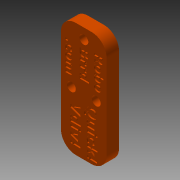
# Autodesk Inventor part: quickvdiv_v1
Saved by Autodesk Inventor 2014 SP1 (Build 180222100, 222)
## iProperties
Created: 2014-02-28
Part Number: quickvdiv_v1
Material: Generic
Document SubType Name: Modeling
Designer: Erin
Density: 1 g/cm^3
Appearance: Default
Author: Erin
Autodesk Inventor part; units mm, degrees
(part 1 of 3)
ref_plane "YZ Plane" through (0, 0, 0) normal (1, 0, 0) x (0, 1, 0)
ref_plane "XY Plane" through (0, 0, 0) normal (0, 0, 1) x (1, 0, 0)
sketch "Sketch1" plane through (0, 0, 0) normal (0, 1, 0) x (-1, 0, 0)
  line L0 (14.5843, 32.1144) -> (14.5843, -2.0167)
  line L1 (0.2969, 32.1144) -> (0.2969, -2.0167)
  line L2 (10.6156, 36.0831) -> (4.2656, 36.0831)
  spline S0 degree 3 poles (14.5843, -2.0167) (14.5843, -4.2083) (12.8073, -5.9854) (10.6156, -5.9854) knots 0 0 0 0 1 1 1 1
  line L3 (14.5843, -2.0167) -> (14.5843, -4.2083) construction
  line L4 (14.5843, -4.2083) -> (12.8073, -5.9854) construction
  line L5 (12.8073, -5.9854) -> (10.6156, -5.9854) construction
  spline S1 degree 3 poles (10.6156, 36.0831) (12.8073, 36.0831) (14.5843, 34.3062) (14.5843, 32.1144) knots 0 0 0 0 1 1 1 1
  line L6 (10.6156, 36.0831) -> (12.8073, 36.0831) construction
  line L7 (12.8073, 36.0831) -> (14.5843, 34.3062) construction
  line L8 (14.5843, 34.3062) -> (14.5843, 32.1144) construction
  spline S2 degree 3 poles (0.2969, 32.1144) (0.2969, 34.3062) (2.0738, 36.0831) (4.2656, 36.0831) knots 0 0 0 0 1 1 1 1
  line L9 (0.2969, 32.1144) -> (0.2969, 34.3062) construction
  line L10 (0.2969, 34.3062) -> (2.0738, 36.0831) construction
  line L11 (2.0738, 36.0831) -> (4.2656, 36.0831) construction
  spline S3 degree 3 poles (4.2656, -5.9854) (2.0738, -5.9854) (0.2969, -4.2083) (0.2969, -2.0167) knots 0 0 0 0 1 1 1 1
  line L12 (4.2656, -5.9854) -> (2.0738, -5.9854) construction
  line L13 (2.0738, -5.9854) -> (0.2969, -4.2083) construction
  line L14 (0.2969, -4.2083) -> (0.2969, -2.0167) construction
  line L15 (4.2656, -5.9854) -> (10.6156, -5.9854)
  spline S4 degree 3 poles (7.1231, 12.2708) (7.1231, 12.826) (6.6728, 13.2762) (6.1176, 13.2762) knots 0 0 0 0 1 1 1 1
  line L16 (7.1231, 12.2708) -> (7.1231, 12.826) construction
  line L17 (7.1231, 12.826) -> (6.6728, 13.2762) construction
  line L18 (6.6728, 13.2762) -> (6.1176, 13.2762) construction
  spline S5 degree 3 poles (6.1176, 13.2762) (5.5624, 13.2762) (5.1122, 12.826) (5.1122, 12.2708) knots 0 0 0 0 1 1 1 1
  line L19 (6.1176, 13.2762) -> (5.5624, 13.2762) construction
  line L20 (5.5624, 13.2762) -> (5.1122, 12.826) construction
  line L21 (5.1122, 12.826) -> (5.1122, 12.2708) construction
  spline S6 degree 3 poles (5.1122, 12.2708) (5.1122, 11.7155) (5.5624, 11.2654) (6.1176, 11.2654) knots 0 0 0 0 1 1 1 1
  line L22 (5.1122, 12.2708) -> (5.1122, 11.7155) construction
  line L23 (5.1122, 11.7155) -> (5.5624, 11.2654) construction
  line L24 (5.5624, 11.2654) -> (6.1176, 11.2654) construction
  spline S7 degree 3 poles (6.1176, 11.2654) (6.6728, 11.2654) (7.1231, 11.7155) (7.1231, 12.2708) knots 0 0 0 0 1 1 1 1
  line L25 (6.1176, 11.2654) -> (6.6728, 11.2654) construction
  line L26 (6.6728, 11.2654) -> (7.1231, 11.7155) construction
  line L27 (7.1231, 11.7155) -> (7.1231, 12.2708) construction
  spline S8 degree 3 poles (9.7689, 12.2708) (9.7689, 12.826) (9.3186, 13.2762) (8.7634, 13.2762) knots 0 0 0 0 1 1 1 1
  line L28 (9.7689, 12.2708) -> (9.7689, 12.826) construction
  line L29 (9.7689, 12.826) -> (9.3186, 13.2762) construction
  line L30 (9.3186, 13.2762) -> (8.7634, 13.2762) construction
  spline S9 degree 3 poles (8.7634, 13.2762) (8.2082, 13.2762) (7.758, 12.826) (7.758, 12.2708) knots 0 0 0 0 1 1 1 1
  line L31 (8.7634, 13.2762) -> (8.2082, 13.2762) construction
  line L32 (8.2082, 13.2762) -> (7.758, 12.826) construction
  line L33 (7.758, 12.826) -> (7.758, 12.2708) construction
  spline S10 degree 3 poles (7.758, 12.2708) (7.758, 11.7155) (8.2082, 11.2654) (8.7634, 11.2654) knots 0 0 0 0 1 1 1 1
  line L34 (7.758, 12.2708) -> (7.758, 11.7155) construction
  line L35 (7.758, 11.7155) -> (8.2082, 11.2654) construction
  line L36 (8.2082, 11.2654) -> (8.7634, 11.2654) construction
  spline S11 degree 3 poles (8.7634, 11.2654) (9.3186, 11.2654) (9.7689, 11.7155) (9.7689, 12.2708) knots 0 0 0 0 1 1 1 1
  line L37 (8.7634, 11.2654) -> (9.3186, 11.2654) construction
  line L38 (9.3186, 11.2654) -> (9.7689, 11.7155) construction
  line L39 (9.7689, 11.7155) -> (9.7689, 12.2708) construction
  spline S12 degree 3 poles (9.7689, 17.5624) (9.7689, 18.1176) (9.3186, 18.5678) (8.7634, 18.5678) knots 0 0 0 0 1 1 1 1
  line L40 (9.7689, 17.5624) -> (9.7689, 18.1176) construction
  line L41 (9.7689, 18.1176) -> (9.3186, 18.5678) construction
  line L42 (9.3186, 18.5678) -> (8.7634, 18.5678) construction
  spline S13 degree 3 poles (8.7634, 18.5678) (8.2082, 18.5678) (7.758, 18.1176) (7.758, 17.5624) knots 0 0 0 0 1 1 1 1
  line L43 (8.7634, 18.5678) -> (8.2082, 18.5678) construction
  line L44 (8.2082, 18.5678) -> (7.758, 18.1176) construction
  line L45 (7.758, 18.1176) -> (7.758, 17.5624) construction
  spline S14 degree 3 poles (7.758, 17.5624) (7.758, 17.0072) (8.2082, 16.557) (8.7634, 16.557) knots 0 0 0 0 1 1 1 1
  line L46 (7.758, 17.5624) -> (7.758, 17.0072) construction
  line L47 (7.758, 17.0072) -> (8.2082, 16.557) construction
  line L48 (8.2082, 16.557) -> (8.7634, 16.557) construction
  spline S15 degree 3 poles (8.7634, 16.557) (9.3186, 16.557) (9.7689, 17.0072) (9.7689, 17.5624) knots 0 0 0 0 1 1 1 1
  line L49 (8.7634, 16.557) -> (9.3186, 16.557) construction
  line L50 (9.3186, 16.557) -> (9.7689, 17.0072) construction
  line L51 (9.7689, 17.0072) -> (9.7689, 17.5624) construction
  spline S16 degree 3 poles (7.1231, 17.5624) (7.1231, 18.1176) (6.6728, 18.5678) (6.1176, 18.5678) knots 0 0 0 0 1 1 1 1
  line L52 (7.1231, 17.5624) -> (7.1231, 18.1176) construction
  line L53 (7.1231, 18.1176) -> (6.6728, 18.5678) construction
  line L54 (6.6728, 18.5678) -> (6.1176, 18.5678) construction
  spline S17 degree 3 poles (6.1176, 18.5678) (5.5624, 18.5678) (5.1122, 18.1176) (5.1122, 17.5624) knots 0 0 0 0 1 1 1 1
  line L55 (6.1176, 18.5678) -> (5.5624, 18.5678) construction
  line L56 (5.5624, 18.5678) -> (5.1122, 18.1176) construction
  line L57 (5.1122, 18.1176) -> (5.1122, 17.5624) construction
  spline S18 degree 3 poles (5.1122, 17.5624) (5.1122, 17.0072) (5.5624, 16.557) (6.1176, 16.557) knots 0 0 0 0 1 1 1 1
  line L58 (5.1122, 17.5624) -> (5.1122, 17.0072) construction
  line L59 (5.1122, 17.0072) -> (5.5624, 16.557) construction
  line L60 (5.5624, 16.557) -> (6.1176, 16.557) construction
  spline S19 degree 3 poles (6.1176, 16.557) (6.6728, 16.557) (7.1231, 17.0072) (7.1231, 17.5624) knots 0 0 0 0 1 1 1 1
  line L61 (6.1176, 16.557) -> (6.6728, 16.557) construction
  line L62 (6.6728, 16.557) -> (7.1231, 17.0072) construction
  line L63 (7.1231, 17.0072) -> (7.1231, 17.5624) construction
  spline S20 degree 3 poles (7.1231, 14.9166) (7.1231, 15.4718) (6.6728, 15.922) (6.1176, 15.922) knots 0 0 0 0 1 1 1 1
  line L64 (7.1231, 14.9166) -> (7.1231, 15.4718) construction
  line L65 (7.1231, 15.4718) -> (6.6728, 15.922) construction
  line L66 (6.6728, 15.922) -> (6.1176, 15.922) construction
  spline S21 degree 3 poles (6.1176, 15.922) (5.5624, 15.922) (5.1122, 15.4718) (5.1122, 14.9166) knots 0 0 0 0 1 1 1 1
  line L67 (6.1176, 15.922) -> (5.5624, 15.922) construction
  line L68 (5.5624, 15.922) -> (5.1122, 15.4718) construction
  line L69 (5.1122, 15.4718) -> (5.1122, 14.9166) construction
  spline S22 degree 3 poles (5.1122, 14.9166) (5.1122, 14.3614) (5.5624, 13.9112) (6.1176, 13.9112) knots 0 0 0 0 1 1 1 1
  line L70 (5.1122, 14.9166) -> (5.1122, 14.3614) construction
  line L71 (5.1122, 14.3614) -> (5.5624, 13.9112) construction
  line L72 (5.5624, 13.9112) -> (6.1176, 13.9112) construction
  spline S23 degree 3 poles (6.1176, 13.9112) (6.6728, 13.9112) (7.1231, 14.3614) (7.1231, 14.9166) knots 0 0 0 0 1 1 1 1
  line L73 (6.1176, 13.9112) -> (6.6728, 13.9112) construction
  line L74 (6.6728, 13.9112) -> (7.1231, 14.3614) construction
  line L75 (7.1231, 14.3614) -> (7.1231, 14.9166) construction
  spline S24 degree 3 poles (9.7689, 14.9166) (9.7689, 15.4718) (9.3186, 15.922) (8.7634, 15.922) knots 0 0 0 0 1 1 1 1
  line L76 (9.7689, 14.9166) -> (9.7689, 15.4718) construction
  line L77 (9.7689, 15.4718) -> (9.3186, 15.922) construction
  line L78 (9.3186, 15.922) -> (8.7634, 15.922) construction
  spline S25 degree 3 poles (8.7634, 15.922) (8.2082, 15.922) (7.758, 15.4718) (7.758, 14.9166) knots 0 0 0 0 1 1 1 1
  line L79 (8.7634, 15.922) -> (8.2082, 15.922) construction
  line L80 (8.2082, 15.922) -> (7.758, 15.4718) construction
  line L81 (7.758, 15.4718) -> (7.758, 14.9166) construction
  spline S26 degree 3 poles (7.758, 14.9166) (7.758, 14.3614) (8.2082, 13.9112) (8.7634, 13.9112) knots 0 0 0 0 1 1 1 1
  line L82 (7.758, 14.9166) -> (7.758, 14.3614) construction
  line L83 (7.758, 14.3614) -> (8.2082, 13.9112) construction
  line L84 (8.2082, 13.9112) -> (8.7634, 13.9112) construction
  spline S27 degree 3 poles (8.7634, 13.9112) (9.3186, 13.9112) (9.7689, 14.3614) (9.7689, 14.9166) knots 0 0 0 0 1 1 1 1
  line L85 (8.7634, 13.9112) -> (9.3186, 13.9112) construction
  line L86 (9.3186, 13.9112) -> (9.7689, 14.3614) construction
  line L87 (9.7689, 14.3614) -> (9.7689, 14.9166) construction
  spline S28 degree 3 poles (7.1231, 1.6875) (7.1231, 2.2427) (6.6728, 2.6929) (6.1176, 2.6929) knots 0 0 0 0 1 1 1 1
  line L88 (7.1231, 1.6875) -> (7.1231, 2.2427) construction
  line L89 (7.1231, 2.2427) -> (6.6728, 2.6929) construction
  line L90 (6.6728, 2.6929) -> (6.1176, 2.6929) construction
  spline S29 degree 3 poles (6.1176, 2.6929) (5.5624, 2.6929) (5.1122, 2.2427) (5.1122, 1.6875) knots 0 0 0 0 1 1 1 1
  line L91 (6.1176, 2.6929) -> (5.5624, 2.6929) construction
  line L92 (5.5624, 2.6929) -> (5.1122, 2.2427) construction
  line L93 (5.1122, 2.2427) -> (5.1122, 1.6875) construction
  spline S30 degree 3 poles (5.1122, 1.6875) (5.1122, 1.1323) (5.5624, 0.6821) (6.1176, 0.6821) knots 0 0 0 0 1 1 1 1
  line L94 (5.1122, 1.6875) -> (5.1122, 1.1323) construction
  line L95 (5.1122, 1.1323) -> (5.5624, 0.6821) construction
  line L96 (5.5624, 0.6821) -> (6.1176, 0.6821) construction
  spline S31 degree 3 poles (6.1176, 0.6821) (6.6728, 0.6821) (7.1231, 1.1323) (7.1231, 1.6875) knots 0 0 0 0 1 1 1 1
  line L97 (6.1176, 0.6821) -> (6.6728, 0.6821) construction
  line L98 (6.6728, 0.6821) -> (7.1231, 1.1323) construction
  line L99 (7.1231, 1.1323) -> (7.1231, 1.6875) construction
  spline S32 degree 3 poles (9.7689, 1.6875) (9.7689, 2.2427) (9.3186, 2.6929) (8.7634, 2.6929) knots 0 0 0 0 1 1 1 1
  line L100 (9.7689, 1.6875) -> (9.7689, 2.2427) construction
  line L101 (9.7689, 2.2427) -> (9.3186, 2.6929) construction
  line L102 (9.3186, 2.6929) -> (8.7634, 2.6929) construction
  spline S33 degree 3 poles (8.7634, 2.6929) (8.2082, 2.6929) (7.758, 2.2427) (7.758, 1.6875) knots 0 0 0 0 1 1 1 1
  line L103 (8.7634, 2.6929) -> (8.2082, 2.6929) construction
  line L104 (8.2082, 2.6929) -> (7.758, 2.2427) construction
  line L105 (7.758, 2.2427) -> (7.758, 1.6875) construction
  spline S34 degree 3 poles (7.758, 1.6875) (7.758, 1.1323) (8.2082, 0.6821) (8.7634, 0.6821) knots 0 0 0 0 1 1 1 1
  line L106 (7.758, 1.6875) -> (7.758, 1.1323) construction
  line L107 (7.758, 1.1323) -> (8.2082, 0.6821) construction
  line L108 (8.2082, 0.6821) -> (8.7634, 0.6821) construction
  spline S35 degree 3 poles (8.7634, 0.6821) (9.3186, 0.6821) (9.7689, 1.1323) (9.7689, 1.6875) knots 0 0 0 0 1 1 1 1
  line L109 (8.7634, 0.6821) -> (9.3186, 0.6821) construction
  line L110 (9.3186, 0.6821) -> (9.7689, 1.1323) construction
  line L111 (9.7689, 1.1323) -> (9.7689, 1.6875) construction
  spline S36 degree 3 poles (7.1231, 30.7915) (7.1231, 31.3467) (6.6728, 31.7969) (6.1176, 31.7969) knots 0 0 0 0 1 1 1 1
  line L112 (7.1231, 30.7915) -> (7.1231, 31.3467) construction
  line L113 (7.1231, 31.3467) -> (6.6728, 31.7969) construction
  line L114 (6.6728, 31.7969) -> (6.1176, 31.7969) construction
  spline S37 degree 3 poles (6.1176, 31.7969) (5.5624, 31.7969) (5.1122, 31.3467) (5.1122, 30.7915) knots 0 0 0 0 1 1 1 1
  line L115 (6.1176, 31.7969) -> (5.5624, 31.7969) construction
  line L116 (5.5624, 31.7969) -> (5.1122, 31.3467) construction
  line L117 (5.1122, 31.3467) -> (5.1122, 30.7915) construction
  spline S38 degree 3 poles (5.1122, 30.7915) (5.1122, 30.2363) (5.5624, 29.7861) (6.1176, 29.7861) knots 0 0 0 0 1 1 1 1
  line L118 (5.1122, 30.7915) -> (5.1122, 30.2363) construction
  line L119 (5.1122, 30.2363) -> (5.5624, 29.7861) construction
  line L120 (5.5624, 29.7861) -> (6.1176, 29.7861) construction
  spline S39 degree 3 poles (6.1176, 29.7861) (6.6728, 29.7861) (7.1231, 30.2363) (7.1231, 30.7915) knots 0 0 0 0 1 1 1 1
  line L121 (6.1176, 29.7861) -> (6.6728, 29.7861) construction
  line L122 (6.6728, 29.7861) -> (7.1231, 30.2363) construction
  line L123 (7.1231, 30.2363) -> (7.1231, 30.7915) construction
  spline S40 degree 3 poles (9.7689, 30.7915) (9.7689, 31.3467) (9.3186, 31.7969) (8.7634, 31.7969) knots 0 0 0 0 1 1 1 1
  line L124 (9.7689, 30.7915) -> (9.7689, 31.3467) construction
  line L125 (9.7689, 31.3467) -> (9.3186, 31.7969) construction
  line L126 (9.3186, 31.7969) -> (8.7634, 31.7969) construction
  spline S41 degree 3 poles (8.7634, 31.7969) (8.2082, 31.7969) (7.758, 31.3467) (7.758, 30.7915) knots 0 0 0 0 1 1 1 1
  line L127 (8.7634, 31.7969) -> (8.2082, 31.7969) construction
  line L128 (8.2082, 31.7969) -> (7.758, 31.3467) construction
  line L129 (7.758, 31.3467) -> (7.758, 30.7915) construction
  spline S42 degree 3 poles (7.758, 30.7915) (7.758, 30.2363) (8.2082, 29.7861) (8.7634, 29.7861) knots 0 0 0 0 1 1 1 1
  line L130 (7.758, 30.7915) -> (7.758, 30.2363) construction
  line L131 (7.758, 30.2363) -> (8.2082, 29.7861) construction
  line L132 (8.2082, 29.7861) -> (8.7634, 29.7861) construction
  spline S43 degree 3 poles (8.7634, 29.7861) (9.3186, 29.7861) (9.7689, 30.2363) (9.7689, 30.7915) knots 0 0 0 0 1 1 1 1
  line L133 (8.7634, 29.7861) -> (9.3186, 29.7861) construction
  line L134 (9.3186, 29.7861) -> (9.7689, 30.2363) construction
  line L135 (9.7689, 30.2363) -> (9.7689, 30.7915) construction
  spline S44 degree 3 poles (9.7689, 28.1457) (9.7689, 28.7009) (9.3186, 29.1511) (8.7634, 29.1511) knots 0 0 0 0 1 1 1 1
  line L136 (9.7689, 28.1457) -> (9.7689, 28.7009) construction
  line L137 (9.7689, 28.7009) -> (9.3186, 29.1511) construction
  line L138 (9.3186, 29.1511) -> (8.7634, 29.1511) construction
  spline S45 degree 3 poles (8.7634, 29.1511) (8.2082, 29.1511) (7.758, 28.7009) (7.758, 28.1457) knots 0 0 0 0 1 1 1 1
  line L139 (8.7634, 29.1511) -> (8.2082, 29.1511) construction
  line L140 (8.2082, 29.1511) -> (7.758, 28.7009) construction
  line L141 (7.758, 28.7009) -> (7.758, 28.1457) construction
  spline S46 degree 3 poles (7.758, 28.1457) (7.758, 27.5904) (8.2082, 27.1403) (8.7634, 27.1403) knots 0 0 0 0 1 1 1 1
  line L142 (7.758, 28.1457) -> (7.758, 27.5904) construction
  line L143 (7.758, 27.5904) -> (8.2082, 27.1403) construction
  line L144 (8.2082, 27.1403) -> (8.7634, 27.1403) construction
  spline S47 degree 3 poles (8.7634, 27.1403) (9.3186, 27.1403) (9.7689, 27.5904) (9.7689, 28.1457) knots 0 0 0 0 1 1 1 1
  line L145 (8.7634, 27.1403) -> (9.3186, 27.1403) construction
  line L146 (9.3186, 27.1403) -> (9.7689, 27.5904) construction
  line L147 (9.7689, 27.5904) -> (9.7689, 28.1457) construction
  spline S48 degree 3 poles (7.1231, 28.1457) (7.1231, 28.7009) (6.6728, 29.1511) (6.1176, 29.1511) knots 0 0 0 0 1 1 1 1
  line L148 (7.1231, 28.1457) -> (7.1231, 28.7009) construction
  line L149 (7.1231, 28.7009) -> (6.6728, 29.1511) construction
  line L150 (6.6728, 29.1511) -> (6.1176, 29.1511) construction
  spline S49 degree 3 poles (6.1176, 29.1511) (5.5624, 29.1511) (5.1122, 28.7009) (5.1122, 28.1457) knots 0 0 0 0 1 1 1 1
  line L151 (6.1176, 29.1511) -> (5.5624, 29.1511) construction
  line L152 (5.5624, 29.1511) -> (5.1122, 28.7009) construction
  line L153 (5.1122, 28.7009) -> (5.1122, 28.1457) construction
  spline S50 degree 3 poles (5.1122, 28.1457) (5.1122, 27.5904) (5.5624, 27.1403) (6.1176, 27.1403) knots 0 0 0 0 1 1 1 1
  line L154 (5.1122, 28.1457) -> (5.1122, 27.5904) construction
  line L155 (5.1122, 27.5904) -> (5.5624, 27.1403) construction
  line L156 (5.5624, 27.1403) -> (6.1176, 27.1403) construction
  spline S51 degree 3 poles (6.1176, 27.1403) (6.6728, 27.1403) (7.1231, 27.5904) (7.1231, 28.1457) knots 0 0 0 0 1 1 1 1
  line L157 (6.1176, 27.1403) -> (6.6728, 27.1403) construction
  line L158 (6.6728, 27.1403) -> (7.1231, 27.5904) construction
  line L159 (7.1231, 27.5904) -> (7.1231, 28.1457) construction
  spline S52 degree 3 poles (7.1231, -0.9584) (7.1231, -0.4031) (6.6728, 0.0471) (6.1176, 0.0471) knots 0 0 0 0 1 1 1 1
  line L160 (7.1231, -0.9584) -> (7.1231, -0.4031) construction
  line L161 (7.1231, -0.4031) -> (6.6728, 0.0471) construction
  line L162 (6.6728, 0.0471) -> (6.1176, 0.0471) construction
  spline S53 degree 3 poles (6.1176, 0.0471) (5.5624, 0.0471) (5.1122, -0.4031) (5.1122, -0.9584) knots 0 0 0 0 1 1 1 1
  line L163 (6.1176, 0.0471) -> (5.5624, 0.0471) construction
  line L164 (5.5624, 0.0471) -> (5.1122, -0.4031) construction
  line L165 (5.1122, -0.4031) -> (5.1122, -0.9584) construction
  spline S54 degree 3 poles (5.1122, -0.9584) (5.1122, -1.5136) (5.5624, -1.9638) (6.1176, -1.9638) knots 0 0 0 0 1 1 1 1
  line L166 (5.1122, -0.9584) -> (5.1122, -1.5136) construction
  line L167 (5.1122, -1.5136) -> (5.5624, -1.9638) construction
  line L168 (5.5624, -1.9638) -> (6.1176, -1.9638) construction
  spline S55 degree 3 poles (6.1176, -1.9638) (6.6728, -1.9638) (7.1231, -1.5136) (7.1231, -0.9584) knots 0 0 0 0 1 1 1 1
  line L169 (6.1176, -1.9638) -> (6.6728, -1.9638) construction
  line L170 (6.6728, -1.9638) -> (7.1231, -1.5136) construction
  line L171 (7.1231, -1.5136) -> (7.1231, -0.9584) construction
  spline S56 degree 3 poles (9.7689, -0.9584) (9.7689, -0.4031) (9.3186, 0.0471) (8.7634, 0.0471) knots 0 0 0 0 1 1 1 1
  line L172 (9.7689, -0.9584) -> (9.7689, -0.4031) construction
  line L173 (9.7689, -0.4031) -> (9.3186, 0.0471) construction
  line L174 (9.3186, 0.0471) -> (8.7634, 0.0471) construction
  spline S57 degree 3 poles (8.7634, 0.0471) (8.2082, 0.0471) (7.758, -0.4031) (7.758, -0.9584) knots 0 0 0 0 1 1 1 1
  line L175 (8.7634, 0.0471) -> (8.2082, 0.0471) construction
  line L176 (8.2082, 0.0471) -> (7.758, -0.4031) construction
  line L177 (7.758, -0.4031) -> (7.758, -0.9584) construction
  spline S58 degree 3 poles (7.758, -0.9584) (7.758, -1.5136) (8.2082, -1.9638) (8.7634, -1.9638) knots 0 0 0 0 1 1 1 1
  line L178 (7.758, -0.9584) -> (7.758, -1.5136) construction
  line L179 (7.758, -1.5136) -> (8.2082, -1.9638) construction
  line L180 (8.2082, -1.9638) -> (8.7634, -1.9638) construction
  spline S59 degree 3 poles (8.7634, -1.9638) (9.3186, -1.9638) (9.7689, -1.5136) (9.7689, -0.9584) knots 0 0 0 0 1 1 1 1
  line L181 (8.7634, -1.9638) -> (9.3186, -1.9638) construction
  line L182 (9.3186, -1.9638) -> (9.7689, -1.5136) construction
  line L183 (9.7689, -1.5136) -> (9.7689, -0.9584) construction
  spline S60 degree 3 poles (4.4773, -4.3979) (4.4773, -3.8427) (4.027, -3.3925) (3.4718, -3.3925) knots 0 0 0 0 1 1 1 1
  line L184 (4.4773, -4.3979) -> (4.4773, -3.8427) construction
  line L185 (4.4773, -3.8427) -> (4.027, -3.3925) construction
  line L186 (4.027, -3.3925) -> (3.4718, -3.3925) construction
  spline S61 degree 3 poles (3.4718, -3.3925) (2.9165, -3.3925) (2.4664, -3.8427) (2.4664, -4.3979) knots 0 0 0 0 1 1 1 1
  line L187 (3.4718, -3.3925) -> (2.9165, -3.3925) construction
  line L188 (2.9165, -3.3925) -> (2.4664, -3.8427) construction
  line L189 (2.4664, -3.8427) -> (2.4664, -4.3979) construction
  spline S62 degree 3 poles (2.4664, -4.3979) (2.4664, -4.9532) (2.9165, -5.4033) (3.4718, -5.4033) knots 0 0 0 0 1 1 1 1
  line L190 (2.4664, -4.3979) -> (2.4664, -4.9532) construction
  line L191 (2.4664, -4.9532) -> (2.9165, -5.4033) construction
  line L192 (2.9165, -5.4033) -> (3.4718, -5.4033) construction
  spline S63 degree 3 poles (3.4718, -5.4033) (4.027, -5.4033) (4.4773, -4.9532) (4.4773, -4.3979) knots 0 0 0 0 1 1 1 1
  line L193 (3.4718, -5.4033) -> (4.027, -5.4033) construction
  line L194 (4.027, -5.4033) -> (4.4773, -4.9532) construction
  line L195 (4.4773, -4.9532) -> (4.4773, -4.3979) construction
  spline S64 degree 3 poles (7.1231, -4.3979) (7.1231, -3.8427) (6.6728, -3.3925) (6.1176, -3.3925) knots 0 0 0 0 1 1 1 1
  line L196 (7.1231, -4.3979) -> (7.1231, -3.8427) construction
  line L197 (7.1231, -3.8427) -> (6.6728, -3.3925) construction
  line L198 (6.6728, -3.3925) -> (6.1176, -3.3925) construction
  spline S65 degree 3 poles (6.1176, -3.3925) (5.5624, -3.3925) (5.1122, -3.8427) (5.1122, -4.3979) knots 0 0 0 0 1 1 1 1
  line L199 (6.1176, -3.3925) -> (5.5624, -3.3925) construction
  line L200 (5.5624, -3.3925) -> (5.1122, -3.8427) construction
  line L201 (5.1122, -3.8427) -> (5.1122, -4.3979) construction
  spline S66 degree 3 poles (5.1122, -4.3979) (5.1122, -4.9532) (5.5624, -5.4033) (6.1176, -5.4033) knots 0 0 0 0 1 1 1 1
  line L202 (5.1122, -4.3979) -> (5.1122, -4.9532) construction
  line L203 (5.1122, -4.9532) -> (5.5624, -5.4033) construction
  line L204 (5.5624, -5.4033) -> (6.1176, -5.4033) construction
  spline S67 degree 3 poles (6.1176, -5.4033) (6.6728, -5.4033) (7.1231, -4.9532) (7.1231, -4.3979) knots 0 0 0 0 1 1 1 1
  line L205 (6.1176, -5.4033) -> (6.6728, -5.4033) construction
  line L206 (6.6728, -5.4033) -> (7.1231, -4.9532) construction
  line L207 (7.1231, -4.9532) -> (7.1231, -4.3979) construction
  spline S68 degree 3 poles (9.7689, -4.3979) (9.7689, -3.8427) (9.3186, -3.3925) (8.7634, -3.3925) knots 0 0 0 0 1 1 1 1
  line L208 (9.7689, -4.3979) -> (9.7689, -3.8427) construction
  line L209 (9.7689, -3.8427) -> (9.3186, -3.3925) construction
  line L210 (9.3186, -3.3925) -> (8.7634, -3.3925) construction
  spline S69 degree 3 poles (8.7634, -3.3925) (8.2082, -3.3925) (7.758, -3.8427) (7.758, -4.3979) knots 0 0 0 0 1 1 1 1
  line L211 (8.7634, -3.3925) -> (8.2082, -3.3925) construction
  line L212 (8.2082, -3.3925) -> (7.758, -3.8427) construction
  line L213 (7.758, -3.8427) -> (7.758, -4.3979) construction
  spline S70 degree 3 poles (7.758, -4.3979) (7.758, -4.9532) (8.2082, -5.4033) (8.7634, -5.4033) knots 0 0 0 0 1 1 1 1
  line L214 (7.758, -4.3979) -> (7.758, -4.9532) construction
  line L215 (7.758, -4.9532) -> (8.2082, -5.4033) construction
  line L216 (8.2082, -5.4033) -> (8.7634, -5.4033) construction
  spline S71 degree 3 poles (8.7634, -5.4033) (9.3186, -5.4033) (9.7689, -4.9532) (9.7689, -4.3979) knots 0 0 0 0 1 1 1 1
  line L217 (8.7634, -5.4033) -> (9.3186, -5.4033) construction
  line L218 (9.3186, -5.4033) -> (9.7689, -4.9532) construction
  line L219 (9.7689, -4.9532) -> (9.7689, -4.3979) construction
  spline S72 degree 3 poles (12.4148, -4.3979) (12.4148, -3.8427) (11.9645, -3.3925) (11.4092, -3.3925) knots 0 0 0 0 1 1 1 1
  line L220 (12.4148, -4.3979) -> (12.4148, -3.8427) construction
  line L221 (12.4148, -3.8427) -> (11.9645, -3.3925) construction
  line L222 (11.9645, -3.3925) -> (11.4092, -3.3925) construction
  spline S73 degree 3 poles (11.4092, -3.3925) (10.854, -3.3925) (10.4038, -3.8427) (10.4038, -4.3979) knots 0 0 0 0 1 1 1 1
  line L223 (11.4092, -3.3925) -> (10.854, -3.3925) construction
  line L224 (10.854, -3.3925) -> (10.4038, -3.8427) construction
  line L225 (10.4038, -3.8427) -> (10.4038, -4.3979) construction
  spline S74 degree 3 poles (10.4038, -4.3979) (10.4038, -4.9532) (10.854, -5.4033) (11.4092, -5.4033) knots 0 0 0 0 1 1 1 1
  line L226 (10.4038, -4.3979) -> (10.4038, -4.9532) construction
  line L227 (10.4038, -4.9532) -> (10.854, -5.4033) construction
  line L228 (10.854, -5.4033) -> (11.4092, -5.4033) construction
  spline S75 degree 3 poles (11.4092, -5.4033) (11.9645, -5.4033) (12.4148, -4.9532) (12.4148, -4.3979) knots 0 0 0 0 1 1 1 1
  line L229 (11.4092, -5.4033) -> (11.9645, -5.4033) construction
  line L230 (11.9645, -5.4033) -> (12.4148, -4.9532) construction
  line L231 (12.4148, -4.9532) -> (12.4148, -4.3979) construction
  spline S76 degree 3 poles (3.6571, 14.9166) (3.6571, 15.6033) (3.1003, 16.1601) (2.4136, 16.1601) knots 0 0 0 0 1 1 1 1
  line L232 (3.6571, 14.9166) -> (3.6571, 15.6033) construction
  line L233 (3.6571, 15.6033) -> (3.1003, 16.1601) construction
  line L234 (3.1003, 16.1601) -> (2.4136, 16.1601) construction
  spline S77 degree 3 poles (2.4136, 16.1601) (1.7268, 16.1601) (1.17, 15.6033) (1.17, 14.9166) knots 0 0 0 0 1 1 1 1
  line L235 (2.4136, 16.1601) -> (1.7268, 16.1601) construction
  line L236 (1.7268, 16.1601) -> (1.17, 15.6033) construction
  line L237 (1.17, 15.6033) -> (1.17, 14.9166) construction
  spline S78 degree 3 poles (1.17, 14.9166) (1.17, 14.2299) (1.7268, 13.6731) (2.4136, 13.6731) knots 0 0 0 0 1 1 1 1
  line L238 (1.17, 14.9166) -> (1.17, 14.2299) construction
  line L239 (1.17, 14.2299) -> (1.7268, 13.6731) construction
  line L240 (1.7268, 13.6731) -> (2.4136, 13.6731) construction
  spline S79 degree 3 poles (2.4136, 13.6731) (3.1003, 13.6731) (3.6571, 14.2299) (3.6571, 14.9166) knots 0 0 0 0 1 1 1 1
  line L241 (2.4136, 13.6731) -> (3.1003, 13.6731) construction
  line L242 (3.1003, 13.6731) -> (3.6571, 14.2299) construction
  line L243 (3.6571, 14.2299) -> (3.6571, 14.9166) construction
  spline S80 degree 3 poles (13.7111, 14.9166) (13.7111, 15.6033) (13.1543, 16.1601) (12.4676, 16.1601) knots 0 0 0 0 1 1 1 1
  line L244 (13.7111, 14.9166) -> (13.7111, 15.6033) construction
  line L245 (13.7111, 15.6033) -> (13.1543, 16.1601) construction
  line L246 (13.1543, 16.1601) -> (12.4676, 16.1601) construction
  spline S81 degree 3 poles (12.4676, 16.1601) (11.7809, 16.1601) (11.2241, 15.6033) (11.2241, 14.9166) knots 0 0 0 0 1 1 1 1
  line L247 (12.4676, 16.1601) -> (11.7809, 16.1601) construction
  line L248 (11.7809, 16.1601) -> (11.2241, 15.6033) construction
  line L249 (11.2241, 15.6033) -> (11.2241, 14.9166) construction
  spline S82 degree 3 poles (11.2241, 14.9166) (11.2241, 14.2299) (11.7809, 13.6731) (12.4676, 13.6731) knots 0 0 0 0 1 1 1 1
  line L250 (11.2241, 14.9166) -> (11.2241, 14.2299) construction
  line L251 (11.2241, 14.2299) -> (11.7809, 13.6731) construction
  line L252 (11.7809, 13.6731) -> (12.4676, 13.6731) construction
  spline S83 degree 3 poles (12.4676, 13.6731) (13.1543, 13.6731) (13.7111, 14.2299) (13.7111, 14.9166) knots 0 0 0 0 1 1 1 1
  line L253 (12.4676, 13.6731) -> (13.1543, 13.6731) construction
  line L254 (13.1543, 13.6731) -> (13.7111, 14.2299) construction
  line L255 (13.7111, 14.2299) -> (13.7111, 14.9166) construction
  spline S84 degree 3 poles (8.6842, 33.9664) (8.6842, 34.6532) (8.1272, 35.21) (7.4405, 35.21) knots 0 0 0 0 1 1 1 1
  line L256 (8.6842, 33.9664) -> (8.6842, 34.6532) construction
  line L257 (8.6842, 34.6532) -> (8.1272, 35.21) construction
  line L258 (8.1272, 35.21) -> (7.4405, 35.21) construction
  spline S85 degree 3 poles (7.4405, 35.21) (6.7538, 35.21) (6.197, 34.6532) (6.197, 33.9664) knots 0 0 0 0 1 1 1 1
  line L259 (7.4405, 35.21) -> (6.7538, 35.21) construction
  line L260 (6.7538, 35.21) -> (6.197, 34.6532) construction
  line L261 (6.197, 34.6532) -> (6.197, 33.9664) construction
  spline S86 degree 3 poles (6.197, 33.9664) (6.197, 33.2797) (6.7538, 32.7229) (7.4405, 32.7229) knots 0 0 0 0 1 1 1 1
  line L262 (6.197, 33.9664) -> (6.197, 33.2797) construction
  line L263 (6.197, 33.2797) -> (6.7538, 32.7229) construction
  line L264 (6.7538, 32.7229) -> (7.4405, 32.7229) construction
  spline S87 degree 3 poles (7.4405, 32.7229) (8.1272, 32.7229) (8.6842, 33.2797) (8.6842, 33.9664) knots 0 0 0 0 1 1 1 1
  line L265 (7.4405, 32.7229) -> (8.1272, 32.7229) construction
  line L266 (8.1272, 32.7229) -> (8.6842, 33.2797) construction
  line L267 (8.6842, 33.2797) -> (8.6842, 33.9664) construction
  spline S88 degree 3 poles (3.6041, 14.9166) (3.6041, 15.574) (3.071, 16.1072) (2.4136, 16.1072) knots 0 0 0 0 1 1 1 1
  line L268 (3.6041, 14.9166) -> (3.6041, 15.574) construction
  line L269 (3.6041, 15.574) -> (3.071, 16.1072) construction
  line L270 (3.071, 16.1072) -> (2.4136, 16.1072) construction
  spline S89 degree 3 poles (2.4136, 16.1072) (1.7561, 16.1072) (1.2229, 15.574) (1.2229, 14.9166) knots 0 0 0 0 1 1 1 1
  line L271 (2.4136, 16.1072) -> (1.7561, 16.1072) construction
  line L272 (1.7561, 16.1072) -> (1.2229, 15.574) construction
  line L273 (1.2229, 15.574) -> (1.2229, 14.9166) construction
  spline S90 degree 3 poles (1.2229, 14.9166) (1.2229, 14.2592) (1.7561, 13.726) (2.4136, 13.726) knots 0 0 0 0 1 1 1 1
  line L274 (1.2229, 14.9166) -> (1.2229, 14.2592) construction
  line L275 (1.2229, 14.2592) -> (1.7561, 13.726) construction
  line L276 (1.7561, 13.726) -> (2.4136, 13.726) construction
  spline S91 degree 3 poles (2.4136, 13.726) (3.071, 13.726) (3.6041, 14.2592) (3.6041, 14.9166) knots 0 0 0 0 1 1 1 1
  line L277 (2.4136, 13.726) -> (3.071, 13.726) construction
  line L278 (3.071, 13.726) -> (3.6041, 14.2592) construction
  line L279 (3.6041, 14.2592) -> (3.6041, 14.9166) construction
  spline S92 degree 3 poles (13.6583, 14.9166) (13.6583, 15.574) (13.125, 16.1072) (12.4676, 16.1072) knots 0 0 0 0 1 1 1 1
  line L280 (13.6583, 14.9166) -> (13.6583, 15.574) construction
  line L281 (13.6583, 15.574) -> (13.125, 16.1072) construction
  line L282 (13.125, 16.1072) -> (12.4676, 16.1072) construction
  spline S93 degree 3 poles (12.4676, 16.1072) (11.8102, 16.1072) (11.277, 15.574) (11.277, 14.9166) knots 0 0 0 0 1 1 1 1
  line L283 (12.4676, 16.1072) -> (11.8102, 16.1072) construction
  line L284 (11.8102, 16.1072) -> (11.277, 15.574) construction
  line L285 (11.277, 15.574) -> (11.277, 14.9166) construction
  spline S94 degree 3 poles (11.277, 14.9166) (11.277, 14.2592) (11.8102, 13.726) (12.4676, 13.726) knots 0 0 0 0 1 1 1 1
  line L286 (11.277, 14.9166) -> (11.277, 14.2592) construction
  line L287 (11.277, 14.2592) -> (11.8102, 13.726) construction
  line L288 (11.8102, 13.726) -> (12.4676, 13.726) construction
  spline S95 degree 3 poles (12.4676, 13.726) (13.125, 13.726) (13.6583, 14.2592) (13.6583, 14.9166) knots 0 0 0 0 1 1 1 1
  line L289 (12.4676, 13.726) -> (13.125, 13.726) construction
  line L290 (13.125, 13.726) -> (13.6583, 14.2592) construction
  line L291 (13.6583, 14.2592) -> (13.6583, 14.9166) construction
  spline S96 degree 3 poles (8.6312, 33.9664) (8.6312, 34.6239) (8.0979, 35.1571) (7.4405, 35.1571) knots 0 0 0 0 1 1 1 1
  line L292 (8.6312, 33.9664) -> (8.6312, 34.6239) construction
  line L293 (8.6312, 34.6239) -> (8.0979, 35.1571) construction
  line L294 (8.0979, 35.1571) -> (7.4405, 35.1571) construction
  spline S97 degree 3 poles (7.4405, 35.1571) (6.7831, 35.1571) (6.2499, 34.6239) (6.2499, 33.9664) knots 0 0 0 0 1 1 1 1
  line L295 (7.4405, 35.1571) -> (6.7831, 35.1571) construction
  line L296 (6.7831, 35.1571) -> (6.2499, 34.6239) construction
  line L297 (6.2499, 34.6239) -> (6.2499, 33.9664) construction
  spline S98 degree 3 poles (6.2499, 33.9664) (6.2499, 33.309) (6.7831, 32.7759) (7.4405, 32.7759) knots 0 0 0 0 1 1 1 1
  line L298 (6.2499, 33.9664) -> (6.2499, 33.309) construction
  line L299 (6.2499, 33.309) -> (6.7831, 32.7759) construction
  line L300 (6.7831, 32.7759) -> (7.4405, 32.7759) construction
  spline S99 degree 3 poles (7.4405, 32.7759) (8.0979, 32.7759) (8.6312, 33.309) (8.6312, 33.9664) knots 0 0 0 0 1 1 1 1
  line L301 (7.4405, 32.7759) -> (8.0979, 32.7759) construction
  line L302 (8.0979, 32.7759) -> (8.6312, 33.309) construction
  line L303 (8.6312, 33.309) -> (8.6312, 33.9664) construction
  spline S100 degree 3 poles (6.5807, 12.2708) (6.5807, 12.5264) (6.3733, 12.7338) (6.1176, 12.7338) knots 0 0 0 0 1 1 1 1
  line L304 (6.5807, 12.2708) -> (6.5807, 12.5264) construction
  line L305 (6.5807, 12.5264) -> (6.3733, 12.7338) construction
  line L306 (6.3733, 12.7338) -> (6.1176, 12.7338) construction
  spline S101 degree 3 poles (6.1176, 12.7338) (5.862, 12.7338) (5.6547, 12.5264) (5.6547, 12.2708) knots 0 0 0 0 1 1 1 1
  line L307 (6.1176, 12.7338) -> (5.862, 12.7338) construction
  line L308 (5.862, 12.7338) -> (5.6547, 12.5264) construction
  line L309 (5.6547, 12.5264) -> (5.6547, 12.2708) construction
  spline S102 degree 3 poles (5.6547, 12.2708) (5.6547, 12.0151) (5.862, 11.8077) (6.1176, 11.8077) knots 0 0 0 0 1 1 1 1
  line L310 (5.6547, 12.2708) -> (5.6547, 12.0151) construction
  line L311 (5.6547, 12.0151) -> (5.862, 11.8077) construction
  line L312 (5.862, 11.8077) -> (6.1176, 11.8077) construction
  spline S103 degree 3 poles (6.1176, 11.8077) (6.3733, 11.8077) (6.5807, 12.0151) (6.5807, 12.2708) knots 0 0 0 0 1 1 1 1
  line L313 (6.1176, 11.8077) -> (6.3733, 11.8077) construction
  line L314 (6.3733, 11.8077) -> (6.5807, 12.0151) construction
  line L315 (6.5807, 12.0151) -> (6.5807, 12.2708) construction
  spline S104 degree 3 poles (9.2265, 12.2708) (9.2265, 12.5264) (9.0191, 12.7338) (8.7634, 12.7338) knots 0 0 0 0 1 1 1 1
  line L316 (9.2265, 12.2708) -> (9.2265, 12.5264) construction
  line L317 (9.2265, 12.5264) -> (9.0191, 12.7338) construction
  line L318 (9.0191, 12.7338) -> (8.7634, 12.7338) construction
  spline S105 degree 3 poles (8.7634, 12.7338) (8.5078, 12.7338) (8.3005, 12.5264) (8.3005, 12.2708) knots 0 0 0 0 1 1 1 1
  line L319 (8.7634, 12.7338) -> (8.5078, 12.7338) construction
  line L320 (8.5078, 12.7338) -> (8.3005, 12.5264) construction
  line L321 (8.3005, 12.5264) -> (8.3005, 12.2708) construction
  spline S106 degree 3 poles (8.3005, 12.2708) (8.3005, 12.0151) (8.5078, 11.8077) (8.7634, 11.8077) knots 0 0 0 0 1 1 1 1
  line L322 (8.3005, 12.2708) -> (8.3005, 12.0151) construction
  line L323 (8.3005, 12.0151) -> (8.5078, 11.8077) construction
  line L324 (8.5078, 11.8077) -> (8.7634, 11.8077) construction
  spline S107 degree 3 poles (8.7634, 11.8077) (9.0191, 11.8077) (9.2265, 12.0151) (9.2265, 12.2708) knots 0 0 0 0 1 1 1 1
  line L325 (8.7634, 11.8077) -> (9.0191, 11.8077) construction
  line L326 (9.0191, 11.8077) -> (9.2265, 12.0151) construction
  line L327 (9.2265, 12.0151) -> (9.2265, 12.2708) construction
  spline S108 degree 3 poles (9.2265, 17.5624) (9.2265, 17.8181) (9.0191, 18.0255) (8.7634, 18.0255) knots 0 0 0 0 1 1 1 1
  line L328 (9.2265, 17.5624) -> (9.2265, 17.8181) construction
  line L329 (9.2265, 17.8181) -> (9.0191, 18.0255) construction
  line L330 (9.0191, 18.0255) -> (8.7634, 18.0255) construction
  spline S109 degree 3 poles (8.7634, 18.0255) (8.5078, 18.0255) (8.3005, 17.8181) (8.3005, 17.5624) knots 0 0 0 0 1 1 1 1
  line L331 (8.7634, 18.0255) -> (8.5078, 18.0255) construction
  line L332 (8.5078, 18.0255) -> (8.3005, 17.8181) construction
  line L333 (8.3005, 17.8181) -> (8.3005, 17.5624) construction
  spline S110 degree 3 poles (8.3005, 17.5624) (8.3005, 17.3068) (8.5078, 17.0993) (8.7634, 17.0993) knots 0 0 0 0 1 1 1 1
  line L334 (8.3005, 17.5624) -> (8.3005, 17.3068) construction
  line L335 (8.3005, 17.3068) -> (8.5078, 17.0993) construction
  line L336 (8.5078, 17.0993) -> (8.7634, 17.0993) construction
  spline S111 degree 3 poles (8.7634, 17.0993) (9.0191, 17.0993) (9.2265, 17.3068) (9.2265, 17.5624) knots 0 0 0 0 1 1 1 1
  line L337 (8.7634, 17.0993) -> (9.0191, 17.0993) construction
  line L338 (9.0191, 17.0993) -> (9.2265, 17.3068) construction
  line L339 (9.2265, 17.3068) -> (9.2265, 17.5624) construction
  spline S112 degree 3 poles (6.5807, 17.5624) (6.5807, 17.8181) (6.3733, 18.0255) (6.1176, 18.0255) knots 0 0 0 0 1 1 1 1
  line L340 (6.5807, 17.5624) -> (6.5807, 17.8181) construction
  line L341 (6.5807, 17.8181) -> (6.3733, 18.0255) construction
  line L342 (6.3733, 18.0255) -> (6.1176, 18.0255) construction
  spline S113 degree 3 poles (6.1176, 18.0255) (5.862, 18.0255) (5.6547, 17.8181) (5.6547, 17.5624) knots 0 0 0 0 1 1 1 1
  line L343 (6.1176, 18.0255) -> (5.862, 18.0255) construction
  line L344 (5.862, 18.0255) -> (5.6547, 17.8181) construction
  line L345 (5.6547, 17.8181) -> (5.6547, 17.5624) construction
  spline S114 degree 3 poles (5.6547, 17.5624) (5.6547, 17.3068) (5.862, 17.0993) (6.1176, 17.0993) knots 0 0 0 0 1 1 1 1
  line L346 (5.6547, 17.5624) -> (5.6547, 17.3068) construction
  line L347 (5.6547, 17.3068) -> (5.862, 17.0993) construction
  line L348 (5.862, 17.0993) -> (6.1176, 17.0993) construction
  spline S115 degree 3 poles (6.1176, 17.0993) (6.3733, 17.0993) (6.5807, 17.3068) (6.5807, 17.5624) knots 0 0 0 0 1 1 1 1
  line L349 (6.1176, 17.0993) -> (6.3733, 17.0993) construction
  line L350 (6.3733, 17.0993) -> (6.5807, 17.3068) construction
  line L351 (6.5807, 17.3068) -> (6.5807, 17.5624) construction
  spline S116 degree 3 poles (6.5807, 14.9166) (6.5807, 15.1723) (6.3733, 15.3797) (6.1176, 15.3797) knots 0 0 0 0 1 1 1 1
  line L352 (6.5807, 14.9166) -> (6.5807, 15.1723) construction
  line L353 (6.5807, 15.1723) -> (6.3733, 15.3797) construction
  line L354 (6.3733, 15.3797) -> (6.1176, 15.3797) construction
  spline S117 degree 3 poles (6.1176, 15.3797) (5.862, 15.3797) (5.6547, 15.1723) (5.6547, 14.9166) knots 0 0 0 0 1 1 1 1
  line L355 (6.1176, 15.3797) -> (5.862, 15.3797) construction
  line L356 (5.862, 15.3797) -> (5.6547, 15.1723) construction
  line L357 (5.6547, 15.1723) -> (5.6547, 14.9166) construction
  spline S118 degree 3 poles (5.6547, 14.9166) (5.6547, 14.661) (5.862, 14.4535) (6.1176, 14.4535) knots 0 0 0 0 1 1 1 1
  line L358 (5.6547, 14.9166) -> (5.6547, 14.661) construction
  line L359 (5.6547, 14.661) -> (5.862, 14.4535) construction
  line L360 (5.862, 14.4535) -> (6.1176, 14.4535) construction
  spline S119 degree 3 poles (6.1176, 14.4535) (6.3733, 14.4535) (6.5807, 14.661) (6.5807, 14.9166) knots 0 0 0 0 1 1 1 1
  line L361 (6.1176, 14.4535) -> (6.3733, 14.4535) construction
  line L362 (6.3733, 14.4535) -> (6.5807, 14.661) construction
  line L363 (6.5807, 14.661) -> (6.5807, 14.9166) construction
  spline S120 degree 3 poles (9.2265, 14.9166) (9.2265, 15.1723) (9.0191, 15.3797) (8.7634, 15.3797) knots 0 0 0 0 1 1 1 1
  line L364 (9.2265, 14.9166) -> (9.2265, 15.1723) construction
  line L365 (9.2265, 15.1723) -> (9.0191, 15.3797) construction
  line L366 (9.0191, 15.3797) -> (8.7634, 15.3797) construction
  spline S121 degree 3 poles (8.7634, 15.3797) (8.5078, 15.3797) (8.3005, 15.1723) (8.3005, 14.9166) knots 0 0 0 0 1 1 1 1
  line L367 (8.7634, 15.3797) -> (8.5078, 15.3797) construction
  line L368 (8.5078, 15.3797) -> (8.3005, 15.1723) construction
  line L369 (8.3005, 15.1723) -> (8.3005, 14.9166) construction
  spline S122 degree 3 poles (8.3005, 14.9166) (8.3005, 14.661) (8.5078, 14.4535) (8.7634, 14.4535) knots 0 0 0 0 1 1 1 1
  line L370 (8.3005, 14.9166) -> (8.3005, 14.661) construction
  line L371 (8.3005, 14.661) -> (8.5078, 14.4535) construction
  line L372 (8.5078, 14.4535) -> (8.7634, 14.4535) construction
  spline S123 degree 3 poles (8.7634, 14.4535) (9.0191, 14.4535) (9.2265, 14.661) (9.2265, 14.9166) knots 0 0 0 0 1 1 1 1
  line L373 (8.7634, 14.4535) -> (9.0191, 14.4535) construction
  line L374 (9.0191, 14.4535) -> (9.2265, 14.661) construction
  line L375 (9.2265, 14.661) -> (9.2265, 14.9166) construction
  spline S124 degree 3 poles (6.5807, 1.6875) (6.5807, 1.9432) (6.3733, 2.1506) (6.1176, 2.1506) knots 0 0 0 0 1 1 1 1
  line L376 (6.5807, 1.6875) -> (6.5807, 1.9432) construction
  line L377 (6.5807, 1.9432) -> (6.3733, 2.1506) construction
  line L378 (6.3733, 2.1506) -> (6.1176, 2.1506) construction
  spline S125 degree 3 poles (6.1176, 2.1506) (5.862, 2.1506) (5.6547, 1.9432) (5.6547, 1.6875) knots 0 0 0 0 1 1 1 1
  line L379 (6.1176, 2.1506) -> (5.862, 2.1506) construction
  line L380 (5.862, 2.1506) -> (5.6547, 1.9432) construction
  line L381 (5.6547, 1.9432) -> (5.6547, 1.6875) construction
  spline S126 degree 3 poles (5.6547, 1.6875) (5.6547, 1.4319) (5.862, 1.2244) (6.1176, 1.2244) knots 0 0 0 0 1 1 1 1
  line L382 (5.6547, 1.6875) -> (5.6547, 1.4319) construction
  line L383 (5.6547, 1.4319) -> (5.862, 1.2244) construction
  line L384 (5.862, 1.2244) -> (6.1176, 1.2244) construction
  spline S127 degree 3 poles (6.1176, 1.2244) (6.3733, 1.2244) (6.5807, 1.4319) (6.5807, 1.6875) knots 0 0 0 0 1 1 1 1
  line L385 (6.1176, 1.2244) -> (6.3733, 1.2244) construction
  line L386 (6.3733, 1.2244) -> (6.5807, 1.4319) construction
  line L387 (6.5807, 1.4319) -> (6.5807, 1.6875) construction
  spline S128 degree 3 poles (9.2265, 1.6875) (9.2265, 1.9432) (9.0191, 2.1506) (8.7634, 2.1506) knots 0 0 0 0 1 1 1 1
  line L388 (9.2265, 1.6875) -> (9.2265, 1.9432) construction
  line L389 (9.2265, 1.9432) -> (9.0191, 2.1506) construction
  line L390 (9.0191, 2.1506) -> (8.7634, 2.1506) construction
  spline S129 degree 3 poles (8.7634, 2.1506) (8.5078, 2.1506) (8.3005, 1.9432) (8.3005, 1.6875) knots 0 0 0 0 1 1 1 1
  line L391 (8.7634, 2.1506) -> (8.5078, 2.1506) construction
  line L392 (8.5078, 2.1506) -> (8.3005, 1.9432) construction
  line L393 (8.3005, 1.9432) -> (8.3005, 1.6875) construction
  spline S130 degree 3 poles (8.3005, 1.6875) (8.3005, 1.4319) (8.5078, 1.2244) (8.7634, 1.2244) knots 0 0 0 0 1 1 1 1
  line L394 (8.3005, 1.6875) -> (8.3005, 1.4319) construction
  line L395 (8.3005, 1.4319) -> (8.5078, 1.2244) construction
  line L396 (8.5078, 1.2244) -> (8.7634, 1.2244) construction
  spline S131 degree 3 poles (8.7634, 1.2244) (9.0191, 1.2244) (9.2265, 1.4319) (9.2265, 1.6875) knots 0 0 0 0 1 1 1 1
  line L397 (8.7634, 1.2244) -> (9.0191, 1.2244) construction
  line L398 (9.0191, 1.2244) -> (9.2265, 1.4319) construction
  line L399 (9.2265, 1.4319) -> (9.2265, 1.6875) construction
  spline S132 degree 3 poles (6.5807, 30.7915) (6.5807, 31.0472) (6.3733, 31.2546) (6.1176, 31.2546) knots 0 0 0 0 1 1 1 1
  line L400 (6.5807, 30.7915) -> (6.5807, 31.0472) construction
  line L401 (6.5807, 31.0472) -> (6.3733, 31.2546) construction
  line L402 (6.3733, 31.2546) -> (6.1176, 31.2546) construction
  spline S133 degree 3 poles (6.1176, 31.2546) (5.862, 31.2546) (5.6547, 31.0472) (5.6547, 30.7915) knots 0 0 0 0 1 1 1 1
  line L403 (6.1176, 31.2546) -> (5.862, 31.2546) construction
  line L404 (5.862, 31.2546) -> (5.6547, 31.0472) construction
  line L405 (5.6547, 31.0472) -> (5.6547, 30.7915) construction
  spline S134 degree 3 poles (5.6547, 30.7915) (5.6547, 30.5359) (5.862, 30.3284) (6.1176, 30.3284) knots 0 0 0 0 1 1 1 1
  line L406 (5.6547, 30.7915) -> (5.6547, 30.5359) construction
  line L407 (5.6547, 30.5359) -> (5.862, 30.3284) construction
  line L408 (5.862, 30.3284) -> (6.1176, 30.3284) construction
  spline S135 degree 3 poles (6.1176, 30.3284) (6.3733, 30.3284) (6.5807, 30.5359) (6.5807, 30.7915) knots 0 0 0 0 1 1 1 1
  line L409 (6.1176, 30.3284) -> (6.3733, 30.3284) construction
  line L410 (6.3733, 30.3284) -> (6.5807, 30.5359) construction
  line L411 (6.5807, 30.5359) -> (6.5807, 30.7915) construction
  spline S136 degree 3 poles (9.2265, 30.7915) (9.2265, 31.0472) (9.0191, 31.2546) (8.7634, 31.2546) knots 0 0 0 0 1 1 1 1
  line L412 (9.2265, 30.7915) -> (9.2265, 31.0472) construction
  line L413 (9.2265, 31.0472) -> (9.0191, 31.2546) construction
  line L414 (9.0191, 31.2546) -> (8.7634, 31.2546) construction
  spline S137 degree 3 poles (8.7634, 31.2546) (8.5078, 31.2546) (8.3005, 31.0472) (8.3005, 30.7915) knots 0 0 0 0 1 1 1 1
  line L415 (8.7634, 31.2546) -> (8.5078, 31.2546) construction
  line L416 (8.5078, 31.2546) -> (8.3005, 31.0472) construction
  line L417 (8.3005, 31.0472) -> (8.3005, 30.7915) construction
  spline S138 degree 3 poles (8.3005, 30.7915) (8.3005, 30.5359) (8.5078, 30.3284) (8.7634, 30.3284) knots 0 0 0 0 1 1 1 1
  line L418 (8.3005, 30.7915) -> (8.3005, 30.5359) construction
  line L419 (8.3005, 30.5359) -> (8.5078, 30.3284) construction
  line L420 (8.5078, 30.3284) -> (8.7634, 30.3284) construction
  spline S139 degree 3 poles (8.7634, 30.3284) (9.0191, 30.3284) (9.2265, 30.5359) (9.2265, 30.7915) knots 0 0 0 0 1 1 1 1
  line L421 (8.7634, 30.3284) -> (9.0191, 30.3284) construction
  line L422 (9.0191, 30.3284) -> (9.2265, 30.5359) construction
  line L423 (9.2265, 30.5359) -> (9.2265, 30.7915) construction
  spline S140 degree 3 poles (9.2265, 28.1457) (9.2265, 28.4013) (9.0191, 28.6088) (8.7634, 28.6088) knots 0 0 0 0 1 1 1 1
  line L424 (9.2265, 28.1457) -> (9.2265, 28.4013) construction
  line L425 (9.2265, 28.4013) -> (9.0191, 28.6088) construction
  line L426 (9.0191, 28.6088) -> (8.7634, 28.6088) construction
  spline S141 degree 3 poles (8.7634, 28.6088) (8.5078, 28.6088) (8.3005, 28.4013) (8.3005, 28.1457) knots 0 0 0 0 1 1 1 1
  line L427 (8.7634, 28.6088) -> (8.5078, 28.6088) construction
  line L428 (8.5078, 28.6088) -> (8.3005, 28.4013) construction
  line L429 (8.3005, 28.4013) -> (8.3005, 28.1457) construction
  spline S142 degree 3 poles (8.3005, 28.1457) (8.3005, 27.89) (8.5078, 27.6826) (8.7634, 27.6826) knots 0 0 0 0 1 1 1 1
  line L430 (8.3005, 28.1457) -> (8.3005, 27.89) construction
  line L431 (8.3005, 27.89) -> (8.5078, 27.6826) construction
  line L432 (8.5078, 27.6826) -> (8.7634, 27.6826) construction
  spline S143 degree 3 poles (8.7634, 27.6826) (9.0191, 27.6826) (9.2265, 27.89) (9.2265, 28.1457) knots 0 0 0 0 1 1 1 1
  line L433 (8.7634, 27.6826) -> (9.0191, 27.6826) construction
  line L434 (9.0191, 27.6826) -> (9.2265, 27.89) construction
  line L435 (9.2265, 27.89) -> (9.2265, 28.1457) construction
  spline S144 degree 3 poles (6.5807, 28.1457) (6.5807, 28.4013) (6.3733, 28.6088) (6.1176, 28.6088) knots 0 0 0 0 1 1 1 1
  line L436 (6.5807, 28.1457) -> (6.5807, 28.4013) construction
  line L437 (6.5807, 28.4013) -> (6.3733, 28.6088) construction
  line L438 (6.3733, 28.6088) -> (6.1176, 28.6088) construction
  spline S145 degree 3 poles (6.1176, 28.6088) (5.862, 28.6088) (5.6547, 28.4013) (5.6547, 28.1457) knots 0 0 0 0 1 1 1 1
  line L439 (6.1176, 28.6088) -> (5.862, 28.6088) construction
  line L440 (5.862, 28.6088) -> (5.6547, 28.4013) construction
  line L441 (5.6547, 28.4013) -> (5.6547, 28.1457) construction
  spline S146 degree 3 poles (5.6547, 28.1457) (5.6547, 27.89) (5.862, 27.6826) (6.1176, 27.6826) knots 0 0 0 0 1 1 1 1
  line L442 (5.6547, 28.1457) -> (5.6547, 27.89) construction
  line L443 (5.6547, 27.89) -> (5.862, 27.6826) construction
  line L444 (5.862, 27.6826) -> (6.1176, 27.6826) construction
  spline S147 degree 3 poles (6.1176, 27.6826) (6.3733, 27.6826) (6.5807, 27.89) (6.5807, 28.1457) knots 0 0 0 0 1 1 1 1
  line L445 (6.1176, 27.6826) -> (6.3733, 27.6826) construction
  line L446 (6.3733, 27.6826) -> (6.5807, 27.89) construction
  line L447 (6.5807, 27.89) -> (6.5807, 28.1457) construction
  spline S148 degree 3 poles (6.5807, -0.9584) (6.5807, -0.7026) (6.3733, -0.4954) (6.1176, -0.4954) knots 0 0 0 0 1 1 1 1
  line L448 (6.5807, -0.9584) -> (6.5807, -0.7026) construction
  line L449 (6.5807, -0.7026) -> (6.3733, -0.4954) construction
  line L450 (6.3733, -0.4954) -> (6.1176, -0.4954) construction
  spline S149 degree 3 poles (6.1176, -0.4954) (5.862, -0.4954) (5.6547, -0.7026) (5.6547, -0.9584) knots 0 0 0 0 1 1 1 1
  line L451 (6.1176, -0.4954) -> (5.862, -0.4954) construction
  line L452 (5.862, -0.4954) -> (5.6547, -0.7026) construction
  line L453 (5.6547, -0.7026) -> (5.6547, -0.9584) construction
  spline S150 degree 3 poles (5.6547, -0.9584) (5.6547, -1.2141) (5.862, -1.4214) (6.1176, -1.4214) knots 0 0 0 0 1 1 1 1
  line L454 (5.6547, -0.9584) -> (5.6547, -1.2141) construction
  line L455 (5.6547, -1.2141) -> (5.862, -1.4214) construction
  line L456 (5.862, -1.4214) -> (6.1176, -1.4214) construction
  spline S151 degree 3 poles (6.1176, -1.4214) (6.3733, -1.4214) (6.5807, -1.2141) (6.5807, -0.9584) knots 0 0 0 0 1 1 1 1
  line L457 (6.1176, -1.4214) -> (6.3733, -1.4214) construction
  line L458 (6.3733, -1.4214) -> (6.5807, -1.2141) construction
  line L459 (6.5807, -1.2141) -> (6.5807, -0.9584) construction
  spline S152 degree 3 poles (9.2265, -0.9584) (9.2265, -0.7026) (9.0191, -0.4954) (8.7634, -0.4954) knots 0 0 0 0 1 1 1 1
  line L460 (9.2265, -0.9584) -> (9.2265, -0.7026) construction
  line L461 (9.2265, -0.7026) -> (9.0191, -0.4954) construction
  line L462 (9.0191, -0.4954) -> (8.7634, -0.4954) construction
  spline S153 degree 3 poles (8.7634, -0.4954) (8.5078, -0.4954) (8.3005, -0.7026) (8.3005, -0.9584) knots 0 0 0 0 1 1 1 1
  line L463 (8.7634, -0.4954) -> (8.5078, -0.4954) construction
  line L464 (8.5078, -0.4954) -> (8.3005, -0.7026) construction
  line L465 (8.3005, -0.7026) -> (8.3005, -0.9584) construction
  spline S154 degree 3 poles (8.3005, -0.9584) (8.3005, -1.2141) (8.5078, -1.4214) (8.7634, -1.4214) knots 0 0 0 0 1 1 1 1
  line L466 (8.3005, -0.9584) -> (8.3005, -1.2141) construction
  line L467 (8.3005, -1.2141) -> (8.5078, -1.4214) construction
  line L468 (8.5078, -1.4214) -> (8.7634, -1.4214) construction
  spline S155 degree 3 poles (8.7634, -1.4214) (9.0191, -1.4214) (9.2265, -1.2141) (9.2265, -0.9584) knots 0 0 0 0 1 1 1 1
  line L469 (8.7634, -1.4214) -> (9.0191, -1.4214) construction
  line L470 (9.0191, -1.4214) -> (9.2265, -1.2141) construction
  line L471 (9.2265, -1.2141) -> (9.2265, -0.9584) construction
  spline S156 degree 3 poles (3.9348, -4.3979) (3.9348, -4.1422) (3.7274, -3.9349) (3.4718, -3.9349) knots 0 0 0 0 1 1 1 1
  line L472 (3.9348, -4.3979) -> (3.9348, -4.1422) construction
  line L473 (3.9348, -4.1422) -> (3.7274, -3.9349) construction
  line L474 (3.7274, -3.9349) -> (3.4718, -3.9349) construction
  spline S157 degree 3 poles (3.4718, -3.9349) (3.2161, -3.9349) (3.0088, -4.1422) (3.0088, -4.3979) knots 0 0 0 0 1 1 1 1
  line L475 (3.4718, -3.9349) -> (3.2161, -3.9349) construction
  line L476 (3.2161, -3.9349) -> (3.0088, -4.1422) construction